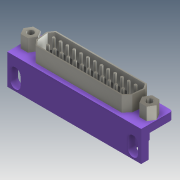
# Autodesk Inventor part: db25-connector-pcb
Saved by Autodesk Inventor 2017 (Build 210142000, 142)
## iProperties
Created: 2018-07-16
Part Number: db25-connector-pcb
Material: Generic
Document SubType Name: Modeling
Designer: Luiz Gustavo
Density: 1 g/cm^3
Appearance: Default
Author: Luiz Gustavo
Autodesk Inventor part; units mm, degrees
ref_plane "YZ Plane" through (0, 0, 0) normal (1, 0, 0) x (0, 1, 0)
ref_plane "XZ Plane" through (0, 0, 0) normal (0, 1, 0) x (-1, 0, 0)
ref_plane "XY Plane" through (0, 0, 0) normal (0, 0, 1) x (1, 0, 0)
sketch "Sketch1" plane through (0, 0, 0) normal (0, 0, 1) x (1, 0, 0)
  line L0 (-26.5, 6.25) -> (26.5, 6.25)
  line L1 (26.5, 6.25) -> (26.5, -6.25)
  line L2 (26.5, -6.25) -> (-26.5, -6.25)
  line L3 (-26.5, -6.25) -> (-26.5, 6.25)
  line L4 (-26.5, 6.25) -> (26.5, -6.25) construction
  line L5 (26.5, 6.25) -> (-26.5, -6.25) construction
  line L6 (-26.5, 0) -> (26.5, 0) construction
  circle A0 centre (-23.5, 0) radius 1.25
  circle A1 centre (-23.5, 0) radius 2.8868 construction
  line L7 (-22.0566, -2.5) -> (-24.9434, 2.5) construction
  line L8 (-26.3868, 0) -> (-20.6132, 0) construction
  line L9 (-22.0566, 2.5) -> (-24.9434, -2.5) construction
  line L10 (-22.0566, 2.5) -> (-24.9434, 2.5)
  line L11 (-24.9434, 2.5) -> (-26.3868, 0)
  line L12 (-24.9434, -2.5) -> (-26.3868, 0)
  line L13 (-22.0566, -2.5) -> (-24.9434, -2.5)
  line L14 (-20.6132, 0) -> (-22.0566, 2.5)
  line L15 (-20.6132, 0) -> (-22.0566, -2.5)
  line L16 (0, 6.25) -> (0, -6.25) construction
  circle A2 centre (23.5, 0) radius 1.25
  line L17 (22.0566, 2.5) -> (24.9434, 2.5)
  line L18 (24.9434, 2.5) -> (26.3868, 0)
  line L19 (24.9434, -2.5) -> (26.3868, 0)
  line L20 (22.0566, -2.5) -> (24.9434, -2.5)
  line L21 (20.6132, 0) -> (22.0566, 2.5)
  line L22 (20.6132, 0) -> (22.0566, -2.5)
  line L23 (-18, 4.5) -> (18, 4.5)
  line L24 (-18, 4.5) -> (-19.5, 2.3)
  line L25 (-19.5, 2.3) -> (-19, -2.3)
  line L26 (-19, -2.3) -> (-17, -4.5)
  line L27 (-17, -4.5) -> (17, -4.5)
  line L28 (17, -4.5) -> (19, -2.3)
  line L29 (19, -2.3) -> (19.5, 2.3)
  line L30 (19.5, 2.3) -> (18, 4.5)
  point P0 (0, 0)
  point P1 (0, 4.5)
  point P2 (0, -4.5)
  dimension "d0" = 53
  dimension "d1" = 12.5
  dimension "d2" = 2.5
  dimension "d4" = 60
  dimension "d5" = 60
  dimension "d6" = 5
  dimension "d7" = 47
  dimension "d8" = 39
  dimension "d9" = 34
  dimension "d10" = 36
  dimension "d11" = 38
  dimension "d12" = 9
  dimension "d13" = 2.2
  dimension "d14" = 2.2
  constraints: 62 end point, 11 midpoint, 9 symmetric about line, 6 point on circle, 5 parallel, 3 centre point, 3 horizontal, 3 point on line, 1 coincident, 1 perpendicular, 2 other
  measures "d0" distance of L1.end L2.end
  measures "d1" distance between parallel lines of L2 L0
  measures "d2" diameter of A0
  measures "d4" angle of L9 L7
  measures "d5" angle of L8 L9
  measures "d6" distance between parallel lines of L13 L10
  measures "d7" distance of A0.centre A2.centre
  measures "d8" distance of L29.end L24.end
  measures "d9" distance of L26.end L27.end
  measures "d10" distance of L23.start L23.end
  measures "d11" distance of L25.end L28.end
  measures "d12" distance between parallel lines of L27 L23
  measures "d13" vertical distance of L27.end L28.end
  measures "d14" vertical distance of L23.end L29.end
extrude "Extrusion1" add sketch "Sketch1" along normal blind 5 contours L14 L15 L13 L12 L11 L10 | L17 L18 L19 L20 L22 L21
extrude "Extrusion2" add sketch "Sketch1" along normal blind 6 contours L23 L30 L29 L28 L27 L26 L25 L24
extrude "Extrusion3" add sketch "Sketch1" against normal blind 12 contours L0 L1 L2 L3 | A0 | L14 L15 L13 L12 L11 L10 | A2 | L17 L18 L19 L20 L22 L21 | L23 L30 L29 L28 L27 L26 L25 L24
sketch "Sketch2" plane through (0, 0, -12) normal (0, 0, -1) x (-1, 0, 0)
  line L0 (26.5, 6.25) -> (-26.5, 6.25) projected
  line L1 (-26.5, 6.25) -> (-26.5, -6.25) projected
  line L2 (-26.5, -6.25) -> (26.5, -6.25) projected
  line L3 (26.5, -6.25) -> (26.5, 6.25) projected
  line L4 (-26.5, 6.25) -> (-26.5, -6.25) projected
  line L5 (-26.5, -3.25) -> (-20, -3.25)
  line L6 (-20, -3.25) -> (-20, 4.25)
  line L7 (-20, 4.25) -> (20, 4.25)
  line L8 (20, 4.25) -> (20, -3.25)
  line L9 (20, -3.25) -> (26.5, -3.25)
  line L10 (0, 6.25) -> (0, -6.25) construction
  line L11 (-26.5, -3.25) -> (-26.5, 6.25)
  line L12 (26.5, 6.25) -> (-26.5, 6.25) projected
  line L13 (-26.5, 6.25) -> (26.5, 6.25)
  line L14 (26.5, 6.25) -> (26.5, -3.25)
  point P0 (0, 0)
  dimension "d21" = 40
  dimension "d22" = 2
  dimension "d23" = 3
  constraints: 18 end point, 4 perpendicular, 4 point on line, 3 collinear, 2 midpoint, 1 other
  measures "d21" distance of L6.end L7.end
  measures "d22" distance between parallel lines of L7 L0
  measures "d23" distance between parallel lines of L2 L9
extrude "Extrusion4" cut sketch "Sketch2" against normal blind 9 contours L3 L9 L8 L7 L6 L5 L1 L0
sketch "Sketch3" plane through (0, 0, 0) normal (0, 1, 0) x (-1, 0, 0)
  line L0 (26.5, -3) -> (26.5, -12) projected
  line L1 (26.5, -12) -> (20, -12) projected
  line L2 (20, -12) -> (20, -3) projected
  arc A0 (23.25, -3.75) -> (21.25, -5.75) centre (23.25, -5.75) ccw
  arc A1 (23.25, -11.25) -> (25.25, -9.25) centre (23.25, -9.25) ccw
  line L3 (23.25, -3.75) -> (23.25, -11.25) construction
  line L4 (25.25, -5.75) -> (25.25, -9.25)
  line L5 (21.25, -9.25) -> (21.25, -5.75)
  line L6 (25.25, -7.5) -> (21.25, -7.5) construction
  line L7 (26.5, -3) -> (20, -3) projected
  arc A2 (21.25, -9.25) -> (23.25, -11.25) centre (23.25, -9.25) ccw
  arc A3 (25.25, -9.25) -> (21.25, -9.25) centre (23.25, -9.25) ccw construction
  arc A4 (25.25, -5.75) -> (23.25, -3.75) centre (23.25, -5.75) ccw
  arc A5 (21.25, -5.75) -> (25.25, -5.75) centre (23.25, -5.75) ccw construction
  line L8 (0, 0) -> (0, -12) construction
  arc A6 (-21.25, -5.75) -> (-23.25, -3.75) centre (-23.25, -5.75) ccw
  arc A7 (-25.25, -9.25) -> (-23.25, -11.25) centre (-23.25, -9.25) ccw
  line L9 (-25.25, -5.75) -> (-25.25, -9.25)
  line L10 (-21.25, -9.25) -> (-21.25, -5.75)
  arc A8 (-23.25, -11.25) -> (-21.25, -9.25) centre (-23.25, -9.25) ccw
  arc A9 (-23.25, -3.75) -> (-25.25, -5.75) centre (-23.25, -5.75) ccw
  dimension "d26" = 4
  dimension "d27" = 7.5
  dimension "d28" = 9
  dimension "d29" = 4.5
  dimension "d30" = 6.5
  dimension "d31" = 3.25
  constraints: 20 point on circle, 14 end point, 10 centre point, 8 symmetric about line, 6 tangent, 2 midpoint, 2 point on line, 2 vertical, 1 equal radius, 1 perpendicular, 4 other
  measures "d26" diameter of A0
  measures "d27" distance of L3.start L3.end
  measures "d28" distance between parallel lines of L7 L1
  measures "d29" distance between parallel lines of L6 L1
  measures "d30" distance between parallel lines of L0 L2
  measures "d31" distance between parallel lines of L0 L3
extrude "Extrusion5" cut sketch "Sketch3" against normal through all contours A4 L4 A1 A2 L5 A0 | L10 A8 A7 L9 A9 A6
sketch "Sketch4" plane through (0, 0, 6) normal (0, 0, 1) x (1, 0, 0)
  line L0 (-16.2, 1.8249) -> (16.2, 1.8249) construction
  circle A0 centre (-16.2, 1.8249) radius 0.5
  circle A1 centre (-13.5, 1.8249) radius 0.5
  circle A2 centre (-10.8, 1.8249) radius 0.5
  circle A3 centre (-8.1, 1.8249) radius 0.5
  circle A4 centre (-5.4, 1.8249) radius 0.5
  circle A5 centre (-2.7, 1.8249) radius 0.5
  circle A6 centre (0, 1.8249) radius 0.5
  circle A7 centre (2.7, 1.8249) radius 0.5
  circle A8 centre (5.4, 1.8249) radius 0.5
  circle A9 centre (8.1, 1.8249) radius 0.5
  circle A10 centre (10.8, 1.8249) radius 0.5
  circle A11 centre (13.5, 1.8249) radius 0.5
  circle A12 centre (16.2, 1.8249) radius 0.5
  line L1 (-14.85, -1.8249) -> (14.85, -1.8249) construction
  circle A13 centre (-14.85, -1.8249) radius 0.5
  circle A14 centre (-12.15, -1.8249) radius 0.5
  circle A15 centre (-9.45, -1.8249) radius 0.5
  circle A16 centre (-6.75, -1.8249) radius 0.5
  circle A17 centre (-4.05, -1.8249) radius 0.5
  circle A18 centre (-1.35, -1.8249) radius 0.5
  circle A19 centre (1.35, -1.8249) radius 0.5
  circle A20 centre (4.05, -1.8249) radius 0.5
  circle A21 centre (6.75, -1.8249) radius 0.5
  circle A22 centre (9.45, -1.8249) radius 0.5
  circle A23 centre (12.15, -1.8249) radius 0.5
  circle A24 centre (14.85, -1.8249) radius 0.5
  line L2 (0, 1.8249) -> (0, -1.8249) construction
  line L3 (18, 4.5) -> (-18, 4.5) construction
  line L4 (-18, 4.5) -> (-19.5, 2.3) construction
  line L5 (-19.5, 2.3) -> (-19, -2.3) construction
  line L6 (-19, -2.3) -> (-17, -4.5) construction
  line L7 (-17, -4.5) -> (17, -4.5) construction
  line L8 (17, -4.5) -> (19, -2.3) construction
  line L9 (19, -2.3) -> (19.5, 2.3) construction
  line L10 (19.5, 2.3) -> (18, 4.5) construction
  line L11 (-17.7357, 4) -> (17.7357, 4)
  line L12 (17.7357, 4) -> (18.983, 2.1707)
  line L13 (18.983, 2.1707) -> (18.5205, -2.0841)
  line L14 (18.5205, -2.0841) -> (16.7788, -4)
  line L15 (16.7788, -4) -> (-16.7788, -4)
  line L16 (-16.7788, -4) -> (-18.5205, -2.0841)
  line L17 (-18.5205, -2.0841) -> (-18.983, 2.1707)
  line L18 (-18.983, 2.1707) -> (-17.7357, 4)
  point P0 (0, 0)
  point P1 (0, 0)
  dimension "d34" = 1
  dimension "d37" = 2.7
  dimension "d44" = 2.7
  dimension "d49" = 0.5
  constraints: 25 centre point, 22 end point, 5 coincident, 4 horizontal, 2 midpoint, 1 equal radius, 1 perpendicular, 53 other
  measures "d34" diameter of A0
  measures "d37" distance of A0.centre A1.centre
  measures "d44" distance of A13.centre A14.centre
  measures "d49" distance between parallel lines of L3 L11
extrude "Extrusion6" cut sketch "Sketch4" against normal up to surface (6 mm away)
fillet "Fillet1" radius 1 4 edges at (-26.5, 6.25, -1.5) (26.5, 6.25, -1.5) (20, 4.25, -7.5) (-20, 4.25, -7.5)
equation "\"d5\" = d4"
equation "\"d14\" = d13"
equation "\"d29\" = 0.5 * d28"
equation "\"d31\" = 0.5 * d30"
equation "\"d44\" = d37"
body "Solid1"
